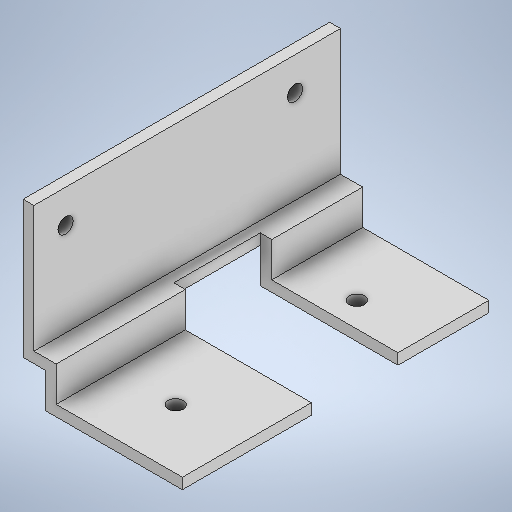
# Autodesk Inventor part: RotaryActBracket
Saved by Autodesk Inventor 2025.1 (Build 291241000, 241)
## iProperties
Created: 2024-11-14
Part Number: RotaryActBracket
Material: Generic
Document SubType Name: Modeling
Designer: hanna
Density: 1 g/cm^3
Appearance: Default
Author: hanna
Autodesk Inventor part; units mm, degrees
ref_plane "YZ Plane" through (0, 0, 0) normal (1, 0, 0) x (0, 1, 0)
ref_plane "XZ Plane" through (0, 0, 0) normal (0, 1, 0) x (-1, 0, 0)
ref_plane "XY Plane" through (0, 0, 0) normal (0, 0, 1) x (1, 0, 0)
sketch "Sketch1" plane through (0, 0, 0) normal (0, 0, 1) x (1, 0, 0)
  line L0 (3, 0) -> (0, 0)
  line L1 (0, 0) -> (0, 9.7)
  line L2 (0, 9.7) -> (-6.163, 9.7)
  line L3 (-6.163, 9.7) -> (-6.163, 47.7)
  line L4 (-6.163, 47.7) -> (-3.163, 47.7)
  line L5 (-3.163, 47.7) -> (-3.163, 12.7)
  line L6 (-3.163, 12.7) -> (3, 12.7)
  line L7 (3, 12.7) -> (3, 3)
  line L8 (3, 3) -> (10.045, 3)
  line L9 (11.5096, 0) -> (9.0351, 0)
  line L10 (10.045, 3) -> (38, 3)
  line L11 (38, 3) -> (38, 0)
  line L12 (0, 0) -> (38, 0)
  point P0 (-3.0815, 9.7)
  dimension "d0" = 9.7
  dimension "d1" = 6.163
  dimension "d2" = 38
  dimension "d3" = 3
  dimension "d6" = 3
  dimension "d7" = 3
  dimension "d8" = 3
  dimension "d10" = 38
  constraints: 26 end point, 8 perpendicular, 4 horizontal, 1 midpoint, 1 point on line
  measures "d0" distance of L0.end L1.end
  measures "d1" distance of L1.end L2.end
  measures "d2" distance of L2.end L3.end
  measures "d3" distance of L3.end L4.end
  measures "d6" vertical distance of point (-3.082, 9.7) L5.end
  measures "d7" distance between parallel lines of L7 L1
  measures "d8" distance from line of L9.start L10
  measures "d10" distance of L11.end L0.end
extrude "Extrusion1" add sketch "Sketch1" along normal blind 85
sketch "Sketch3" plane through (3, 3, 0) normal (1, 0, 0) x (0, 0, -1)
  point P0 (0, -3)
sketch "Sketch8" plane through (-3.163, 12.7, 0) normal (1, 0, 0) x (0, 0, -1)
  circle A0 centre (-76.25, 25.85) radius 2.1
  line L0 (-85, 0) -> (-85, 35) projected
  line L1 (0, 35) -> (-85, 35) projected
  point P0 (0, -12.7)
  dimension "d28" = 4.2
  dimension "d29" = 8.75
  dimension "d30" = 9.15
  constraints: 1 centre point
  measures "d28" diameter of A0
  measures "d29" distance from line of L0 A0.centre
  measures "d30" distance from line of L1 A0.centre
hole "Hole1" at (-3.163, 38.55, 76.25) direction (-1, 0, 0) diameter 4.2 end through all
sketch "Sketch9" plane through (-3.163, 12.7, 0) normal (1, 0, 0) x (0, 0, -1)
  circle A0 centre (-12.601, 25.85) radius 2.1
  line L0 (0, 35) -> (-85, 35) projected
  line L1 (0, 0) -> (0, 35) projected
  point P0 (0, -12.7)
  dimension "d38" = 4.2
  dimension "d39" = 9.15
  dimension "d40" = 12.601
  constraints: 1 centre point
  measures "d38" diameter of A0
  measures "d39" distance from line of L0 A0.centre
  measures "d40" distance from line of L1 A0.centre
hole "Hole2" at (-3.163, 38.55, 12.601) direction (-1, 0, 0) diameter 4.2 end through all
sketch "Sketch10" plane through (0, 0, 0) normal (0, -1, 0) x (1, 0, 0)
  line L0 (38, 0) -> (38, 85) projected
  line L1 (0, 0) -> (0, 85) projected
  line L2 (38, 25.2) -> (0, 25.2)
  line L3 (0, 25.2) -> (0, 49.2)
  line L4 (0, 49.2) -> (38, 49.2)
  line L5 (38, 49.2) -> (38, 25.2)
  line L6 (0, 0) -> (38, 0) projected
  line L7 (0, 85) -> (38, 85) projected
  point P0 (38, 49.2)
  point P1 (0, 25.2)
  dimension "d49" = 24
  dimension "d52" = 35.8
  constraints: 8 end point, 2 parallel, 2 point on line, 1 horizontal, 1 perpendicular
  measures "d49" distance between parallel lines of L4 L2
  measures "d52" distance between parallel lines of L4 L7
extrude "Extrusion7" cut sketch "Sketch10" against normal blind 3 contours L2 L1 L4 L0
sketch "Sketch12" plane through (3, 3, 85) normal (0, 1, 0) x (1, 0, 0)
  circle A0 centre (16.672, 16.473) radius 2.1
  line L0 (35, 0) -> (0, 0) projected
  line L1 (0, 35.8) -> (0, 0) projected
  point P0 (-3, 85)
  dimension "d63" = 4.2
  dimension "d64" = 16.473
  dimension "d65" = 16.672
  constraints: 1 centre point
  measures "d63" diameter of A0
  measures "d64" distance from line of L0 A0.centre
  measures "d65" distance from line of L1 A0.centre
hole "Hole4" at (19.672, 3, 68.527) direction (0, -1, 0) diameter 4.2 end through all
sketch "Sketch13" plane through (3, 3, 0) normal (0, 1, 0) x (1, 0, 0)
  circle A0 centre (16.672, -18.288) radius 2.1
  line L0 (0, 0) -> (0, -25.2) projected
  line L1 (35, 0) -> (0, 0) projected
  point P0 (-3, 0)
  dimension "d73" = 4.2
  dimension "d74" = 16.672
  dimension "d75" = 18.288
  constraints: 1 centre point
  measures "d73" diameter of A0
  measures "d74" distance from line of L0 A0.centre
  measures "d75" distance from line of L1 A0.centre
hole "Hole5" at (19.672, 3, 18.288) direction (0, -1, 0) diameter 4.2 end through all
sketch "Sketch14" plane through (3, 3, 0) normal (1, 0, 0) x (0, 0, -1)
  line L0 (-49.2, 0) -> (-85, 0) projected
  line L1 (0, 9.7) -> (-85, 9.7) projected
  line L2 (-49.2, 0) -> (-25.2, 0)
  line L3 (-25.2, 0) -> (-25.2, 9.7)
  line L4 (-25.2, 9.7) -> (-49.2, 9.7)
  line L5 (-49.2, 9.7) -> (-49.2, 0)
  point P0 (0, -3)
  point P1 (-49.2, 9.7)
  dimension "d83" = 24
  constraints: 8 end point, 2 parallel, 1 horizontal, 1 perpendicular, 1 point on line
  measures "d83" distance of L4.end L3.end
extrude "Extrusion8" cut sketch "Sketch14" against normal blind 3.2
body "Solid1"
